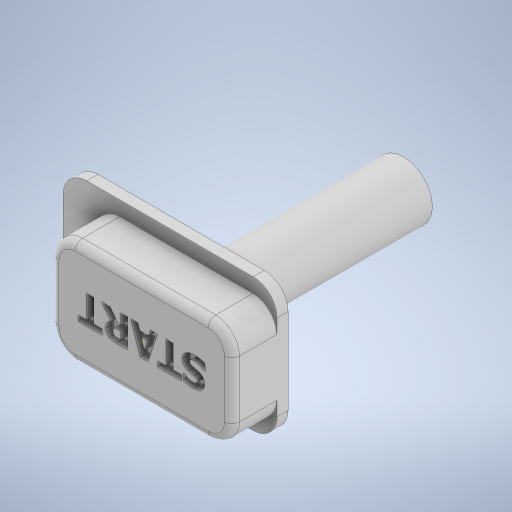
# Autodesk Inventor part: Button Cover
Saved by Autodesk Inventor 2023 (Build 270158000, 158)
## iProperties
Created: 2024-03-21
Part Number: Button Cover
Material: Generic
Document SubType Name: Modeling
Designer: Pobe Tran
Density: 1 g/cm^3
Appearance: Default
Author: Pobe Tran
Autodesk Inventor part; units mm, degrees
ref_plane "YZ Plane" through (0, 0, 0) normal (1, 0, 0) x (0, 1, 0)
ref_plane "XZ Plane" through (0, 0, 0) normal (0, 1, 0) x (-1, 0, 0)
ref_plane "XY Plane" through (0, 0, 0) normal (0, 0, 1) x (1, 0, 0)
sketch "Sketch1" plane through (0, 0, 0) normal (0, 0, 1) x (1, 0, 0)
  circle A0 centre (0, 0) radius 1.75 projected
  circle A1 centre (0, 0) radius 3.85
  point P0 (0, 0)
  constraints: 1 centre point
extrude "Extrusion1" add sketch "Sketch1" against normal blind 5
sketch "Sketch2" plane through (0, 0, 0) normal (0, 0, 1) x (1, 0, 0)
  point P0 (0, 0)
sketch "Sketch3" plane through (0, 0, 0) normal (0, 0, 1) x (1, 0, 0)
  circle A0 centre (0, 0) radius 3.85
  constraints: 1 centre point, 1 coincident
extrude "Extrusion2" add sketch "Sketch3" along normal blind 22.5
sketch "Sketch4" plane through (0, 0, 22.5) normal (0, 0, 1) x (1, 0, 0)
  line L0 (12.065, -6.985) -> (-12.065, -6.985)
  line L1 (-12.065, -6.985) -> (-12.065, 6.985)
  line L2 (-12.065, 6.985) -> (12.065, 6.985)
  line L3 (12.065, 6.985) -> (12.065, -6.985)
  circle A0 centre (0, 0) radius 1.85 projected
  line L4 (12.065, -6.985) -> (-12.065, 6.985) construction
  line L5 (-12.065, -6.985) -> (12.065, 6.985) construction
  line L6 (12.065, 12.065) -> (-12.065, 12.065) construction
  line L7 (-12.065, 12.065) -> (-12.065, 26.035) construction
  line L8 (-12.065, 26.035) -> (12.065, 26.035) construction
  line L9 (12.065, 26.035) -> (12.065, 12.065) construction
  line L10 (12.065, 12.065) -> (-12.065, 26.035) construction
  line L11 (-12.065, 12.065) -> (12.065, 26.035) construction
  line L12 (12.065, -8.89) -> (-16.51, -8.89)
  line L13 (-16.51, -8.89) -> (-16.51, 8.89)
  line L14 (-16.51, 8.89) -> (12.065, 8.89)
  line L15 (16.51, -8.89) -> (-16.51, 8.89) construction
  line L16 (-16.51, -8.89) -> (12.065, 6.4965) construction
  line L17 (12.065, -8.89) -> (12.065, 8.89)
  point P0 (0, 0)
  point P1 (0, 19.05)
  dimension "d6" = 24.13
  dimension "d7" = 13.97
  dimension "d10" = 19.05
  dimension "d16" = 17.78
  constraints: 36 end point, 3 midpoint, 3 parallel, 3 perpendicular, 2 horizontal, 2 point on line, 1 collinear, 1 vertical, 10 other
  measures "d6" distance of L1.end L2.end
  measures "d7" distance of L0.end L1.end
  measures "d10" distance of L0.start L6.start
  measures "d16" distance of L12.end L13.end
extrude "Extrusion3" add sketch "Sketch4" along normal blind 1.5 contours L17 L12 L13 L14 L2 L1 L0 | L0 L1 L2 L3 | A0
extrude "Extrusion4" add sketch "Sketch4" along normal blind 7.5 contours L0 L1 L2 L3 | A0
fillet "Fillet1" radius 3.175 8 edges at (-12.065, 6.985, 27) (12.065, 6.985, 27) (12.065, -6.985, 27) (-12.065, -6.985, 27) (-16.51, -8.89, 23.25) (12.065, 8.89, 23.25) (-16.51, 8.89, 23.25) (12.065, -8.89, 23.25)
sketch "Sketch5" plane through (0, 0, 30) normal (0, 0, 1) x (1, 0, 0)
  point P0 (0, 0)
sketch "Sketch6" plane through (0, 0, 30) normal (0, 0, 1) x (1, 0, 0)
  line L0 (8.6541, -1.9938) -> (-8.6541, -1.9938) construction
  line L1 (-8.6541, -1.9938) -> (-8.6541, 1.9938) construction
  line L2 (-8.6541, 1.9938) -> (8.6541, 1.9938) construction
  line L3 (8.6541, 1.9938) -> (8.6541, -1.9938) construction
  line L4 (-12.065, 3.81) -> (-12.065, -3.81) projected
  line L5 (-8.89, -6.985) -> (8.89, -6.985) projected
  spline S0 degree 2 poles (7.0825, 1.9521) (7.5209, 1.9521) (8.1817, 1.7823) (8.4657, 1.6588) knots 0 0 0 1 2 2 2
  line L6 (8.4657, 1.6588) -> (8.4657, 0.751)
  line L7 (8.4657, 0.751) -> (8.3793, 0.751)
  spline S1 degree 2 poles (8.3793, 0.751) (8.0921, 0.995) (7.4036, 1.2574) (7.0794, 1.2574) knots 0 0 0 1 2 2 2
  spline S2 degree 2 poles (7.0794, 1.2574) (6.9961, 1.2574) (6.7275, 1.2204) (6.6472, 1.1833) knots 0 0 0 1 2 2 2
  spline S3 degree 2 poles (6.6472, 1.1833) (6.5484, 1.1401) (6.4094, 0.9826) (6.4094, 0.856) knots 0 0 0 1 2 2 2
  spline S4 degree 2 poles (6.4094, 0.856) (6.4094, 0.7109) (6.6348, 0.5318) (6.7892, 0.4917) knots 0 0 0 1 2 2 2
  spline S5 degree 2 poles (6.7892, 0.4917) (6.9837, 0.4392) (7.4252, 0.3497) (7.6197, 0.2817) knots 0 0 0 1 2 2 2
  spline S6 degree 2 poles (7.6197, 0.2817) (8.0613, 0.1274) (8.4441, -0.4006) (8.4441, -0.7958) knots 0 0 0 1 2 2 2
  spline S7 degree 2 poles (8.4441, -0.7958) (8.4441, -1.3299) (7.5395, -1.9938) (6.8602, -1.9938) knots 0 0 0 1 2 2 2
  spline S8 degree 2 poles (6.8602, -1.9938) (6.5206, -1.9938) (5.8475, -1.8548) (5.582, -1.7375) knots 0 0 0 1 2 2 2
  line L8 (5.582, -1.7375) -> (5.582, -0.8668)
  line L9 (5.582, -0.8668) -> (5.6653, -0.8668)
  spline S9 degree 2 poles (5.6653, -0.8668) (5.8784, -1.049) (6.4897, -1.2991) (6.8108, -1.2991) knots 0 0 0 1 2 2 2
  spline S10 degree 2 poles (6.8108, -1.2991) (6.9374, -1.2991) (7.135, -1.262) (7.2462, -1.2126) knots 0 0 0 1 2 2 2
  spline S11 degree 2 poles (7.2462, -1.2126) (7.3357, -1.1725) (7.4654, -1.0119) (7.4654, -0.9131) knots 0 0 0 1 2 2 2
  spline S12 degree 2 poles (7.4654, -0.9131) (7.4654, -0.7649) (7.2585, -0.5951) (6.9621, -0.5272) knots 0 0 0 1 2 2 2
  spline S13 degree 2 poles (6.9621, -0.5272) (6.7707, -0.484) (6.4156, -0.4006) (6.2118, -0.3296) knots 0 0 0 1 2 2 2
  spline S14 degree 2 poles (6.2118, -0.3296) (5.8166, -0.1845) (5.4307, 0.2972) (5.4307, 0.6924) knots 0 0 0 1 2 2 2
  spline S15 degree 2 poles (5.4307, 0.6924) (5.4307, 1.2605) (6.323, 1.9521) (7.0825, 1.9521) knots 0 0 0 1 2 2 2
  line L10 (4.208, 1.8842) -> (4.208, -1.2003)
  line L11 (4.208, -1.2003) -> (5.335, -1.2003)
  line L12 (5.335, -1.2003) -> (5.335, -1.9258)
  line L13 (5.335, -1.9258) -> (2.124, -1.9258)
  line L14 (2.124, -1.9258) -> (2.124, -1.2003)
  line L15 (2.124, -1.2003) -> (3.2509, -1.2003)
  line L16 (3.2509, -1.2003) -> (3.2509, 1.8842)
  line L17 (3.2509, 1.8842) -> (4.208, 1.8842)
  line L18 (2.1425, 1.8842) -> (0.855, -1.9258)
  line L19 (0.855, -1.9258) -> (-0.1886, -1.9258)
  line L20 (-0.1886, -1.9258) -> (-1.4761, 1.8842)
  line L21 (-1.4761, 1.8842) -> (-0.4912, 1.8842)
  line L22 (-0.4912, 1.8842) -> (-0.2534, 1.1061)
  line L23 (-0.2534, 1.1061) -> (0.9445, 1.1061)
  line L24 (0.9445, 1.1061) -> (1.1854, 1.8842)
  line L25 (1.1854, 1.8842) -> (2.1425, 1.8842)
  line L26 (-0.0435, 0.4145) -> (0.3455, -0.8452)
  line L27 (0.3455, -0.8452) -> (0.7377, 0.4145)
  line L28 (0.7377, 0.4145) -> (-0.0435, 0.4145)
  line L29 (-5.3756, 1.8842) -> (-4.2116, 1.8842)
  line L30 (-4.2116, 1.8842) -> (-3.1526, 0.4855)
  line L31 (-3.1526, 0.4855) -> (-2.8068, 0.4855)
  line L32 (-2.8068, 0.4855) -> (-2.8068, 1.8842)
  line L33 (-2.8068, 1.8842) -> (-1.8559, 1.8842)
  line L34 (-1.8559, 1.8842) -> (-1.8559, -1.9258)
  line L35 (-1.8559, -1.9258) -> (-3.3873, -1.9258)
  spline S16 degree 2 poles (-3.3873, -1.9258) (-3.7053, -1.9258) (-4.1746, -1.8456) (-4.3753, -1.7221) knots 0 0 0 1 2 2 2
  spline S17 degree 2 poles (-4.3753, -1.7221) (-4.579, -1.5924) (-4.8199, -1.1879) (-4.8199, -0.8792) knots 0 0 0 1 2 2 2
  spline S18 degree 2 poles (-4.8199, -0.8792) (-4.8199, -0.4438) (-4.4247, 0.1027) (-4.0943, 0.2632) knots 0 0 0 1 2 2 2
  line L36 (-4.0943, 0.2632) -> (-5.3756, 1.8842)
  spline S19 degree 2 poles (-3.838, -0.7587) (-3.838, -0.9039) (-3.7269, -1.1107) (-3.6003, -1.1663) knots 0 0 0 1 2 2 2
  spline S20 degree 2 poles (-3.6003, -1.1663) (-3.5108, -1.2034) (-3.2916, -1.225) (-3.1279, -1.225) knots 0 0 0 1 2 2 2
  line L37 (-3.1279, -1.225) -> (-2.8068, -1.225)
  line L38 (-2.8068, -1.225) -> (-2.8068, -0.1999)
  line L39 (-2.8068, -0.1999) -> (-3.0816, -0.1999)
  spline S21 degree 2 poles (-3.0816, -0.1999) (-3.2792, -0.1999) (-3.5602, -0.2493) (-3.6559, -0.3265) knots 0 0 0 1 2 2 2
  spline S22 degree 2 poles (-3.6559, -0.3265) (-3.7485, -0.4006) (-3.838, -0.5982) (-3.838, -0.7587) knots 0 0 0 1 2 2 2
  line L40 (-6.3914, 1.8842) -> (-6.3914, -1.2003)
  line L41 (-6.3914, -1.2003) -> (-5.2645, -1.2003)
  line L42 (-5.2645, -1.2003) -> (-5.2645, -1.9258)
  line L43 (-5.2645, -1.9258) -> (-8.4755, -1.9258)
  line L44 (-8.4755, -1.9258) -> (-8.4755, -1.2003)
  line L45 (-8.4755, -1.2003) -> (-7.3486, -1.2003)
  line L46 (-7.3486, -1.2003) -> (-7.3486, 1.8842)
  line L47 (-7.3486, 1.8842) -> (-6.3914, 1.8842)
  point P0 (0, 0)
  point P1 (-8.6541, 0)
  point P2 (-12.065, 0)
  point P3 (0, -1.9938)
  point P4 (0, -6.985)
  constraints: 4 midpoint, 1 horizontal alignment, 1 vertical alignment, 2 other
emboss "Emboss1" sketch "Sketch6" operation cut depth 1 direction (0, 0, -1)
fillet "Fillet2" radius 1 8 edges at (0, 6.985, 30) (11.1351, 6.0551, 30) (12.065, 0, 30) (11.1351, -6.0551, 30) (0, -6.985, 30) (-11.1351, -6.0551, 30) (-12.065, 0, 30) (-11.1351, 6.0551, 30)
body "Solid1"
